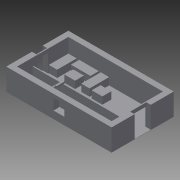
# Autodesk Inventor part: West_Structure_1st_Floor_CAFS
Saved by Autodesk Inventor 2014 (Build 180170000, 170)
## iProperties
Created: 2013-07-10
Part Number: West_Structure_1st_Floor_CAFS
Material: Generic
Document SubType Name: Modeling
Designer: jmw3
Density: 1 g/cm^3
Appearance: Default
Author: jmw3
Autodesk Inventor part; units mm, degrees
ref_plane "YZ Plane" through (0, 0, 0) normal (1, 0, 0) x (0, 1, 0)
ref_plane "XZ Plane" through (0, 0, 0) normal (0, 1, 0) x (-1, 0, 0)
ref_plane "XY Plane" through (0, 0, 0) normal (0, 0, 1) x (1, 0, 0)
sketch "Sketch1" plane through (0, 0, 0) normal (0, 0, 1) x (1, 0, 0)
  line L0 (-8321.04, 0) -> (8321.04, 0) projected
  line L1 (-5943.6, 3505.2) -> (5943.6, 3505.2)
  line L2 (-5334, 2895.6) -> (5334, 2895.6)
  line L3 (-4572, 2895.6) -> (-4419.6, 2895.6)
  line L4 (-1981.2, -2006.6) -> (-4445, -2006.6)
  line L5 (-4445, -2006.6) -> (-4445, -1892.3)
  line L6 (-1219.2, -2895.6) -> (-1066.8, -2895.6)
  line L7 (5334, -2895.6) -> (0, -2895.6)
  line L8 (0, -2895.6) -> (-5334, -2895.6)
  line L9 (5943.6, -3505.2) -> (0, -3505.2)
  line L10 (0, -3505.2) -> (-5943.6, -3505.2)
  line L11 (5334, 914.4) -> (5943.6, 914.4)
  line L12 (5943.6, -914.4) -> (5334, -914.4)
  line L13 (5334, 2895.6) -> (5334, 914.4)
  line L14 (5334, -914.4) -> (5334, -2895.6)
  line L15 (5943.6, 3505.2) -> (5943.6, 914.4)
  line L16 (5943.6, -914.4) -> (5943.6, -3505.2)
  line L17 (-4445, -2006.6) -> (5334, -2006.6)
  line L18 (5334, -1892.3) -> (-4445, -1892.3)
  line L19 (-4445, -1892.3) -> (-4445, -2006.6)
  line L20 (5334, -1892.3) -> (5334, -2006.6)
  line L21 (-5943.6, 609.6) -> (-5334, 609.6)
  line L22 (-5334, -609.6) -> (-5943.6, -609.6)
  line L23 (-5943.6, -3505.2) -> (-5943.6, -609.6)
  line L24 (-5943.6, 609.6) -> (-5943.6, 3505.2)
  line L25 (-5334, -2895.6) -> (-5334, -609.6)
  line L26 (-5334, 609.6) -> (-5334, 2895.6)
  line L27 (-4445, -2006.6) -> (-4419.6, -2006.6)
  line L28 (-4419.6, 2895.6) -> (-4572, 2895.6)
  line L29 (-4445, -1892.3) -> (-4445, -2006.6)
  line L30 (0, -4907.28) -> (0, 4907.28) projected
  dimension "d18" = 7010.4
  dimension "d19" = 609.6
  dimension "d20" = 609.6
  dimension "d23" = 1828.8
  dimension "d24" = 2590.8
  dimension "d25" = 609.6
  dimension "d28" = 114.3
  dimension "d29" = 0
  dimension "d34" = 1219.2
  dimension "d35" = 2895.6
  dimension "d36" = 609.6
  dimension "d46" = 889
  dimension "d105" = 889
  dimension "d106" = 11887.2
  constraints: 58 end point, 17 parallel, 8 horizontal, 7 collinear, 6 perpendicular, 4 point on line, 2 other
  measures "d18" distance between parallel lines of L10 L1
  measures "d19" distance between parallel lines of L10 L8
  measures "d20" distance between parallel lines of L1 L2
  measures "d23" distance between parallel lines of L12 L11
  measures "d24" distance between parallel lines of L9 L12
  measures "d25" distance between parallel lines of L15 L13
  measures "d28" distance between parallel lines of L17 L18
  measures "d29" distance between parallel lines of L13 L20
  measures "d34" distance between parallel lines of L22 L21
  measures "d35" distance between parallel lines of L10 L22
  measures "d36" distance between parallel lines of L24 L26
  measures "d46" distance between parallel lines of L26 L5
  measures "d105" distance from line of L6.end L17
  measures "d106" distance between parallel lines of L15 L24
extrude "Extrusion9" add sketch "Sketch1" along normal blind 2438.4 contours L18 L14 L17 L30 | L30 L17 L4 L5 L18 | L1 L30 L2 L26 L21 L24 | L1 L15 L11 L13 L2 L30 | L14 L12 L16 L9 L30 L7 | L30 L10 L23 L22 L25 L8 L6
sketch "Sketch8" plane through (0, 0, 0) normal (0, 0, -1) x (-1, 0, 0)
  line L0 (5943.6, 3505.2) -> (-5943.6, 3505.2) projected
  line L1 (-5943.6, 3505.2) -> (-5943.6, 914.4) projected
  line L2 (-5943.6, 914.4) -> (-5334, 914.4) projected
  line L3 (-5334, 914.4) -> (-5334, 2895.6) projected
  line L4 (-5334, 2895.6) -> (5334, 2895.6) projected
  line L5 (5334, 2895.6) -> (5334, 609.6) projected
  line L6 (5334, 609.6) -> (5943.6, 609.6) projected
  line L7 (5943.6, 609.6) -> (5943.6, 3505.2) projected
  line L8 (-5943.6, 3505.2) -> (5943.6, 3505.2)
  line L9 (5943.6, 3505.2) -> (5943.6, -3505.2)
  line L10 (5943.6, -3505.2) -> (-5943.6, -3505.2)
  line L11 (-5943.6, -3505.2) -> (-5943.6, 3505.2)
  point P0 (0, 0)
  constraints: 8 end point, 2 parallel, 1 horizontal, 1 perpendicular
extrude "Extrusion10" add sketch "Sketch8" along normal blind 25.4
sketch "Sketch10" plane through (-4445, -2006.6, 2438.4) normal (0, -1, 0) x (1, 0, 0)
  line L0 (0, -2438.4) -> (9779, -2438.4) projected
  line L1 (0, -2438.4) -> (0, 0) projected
  line L2 (723.9, -2438.4) -> (914.4, -2438.4)
  line L3 (914.4, -2438.4) -> (914.4, -2254.25)
  line L4 (914.4, -2254.25) -> (723.9, -2254.25)
  line L5 (723.9, -2254.25) -> (723.9, -2438.4)
  line L6 (914.4, -2254.25) -> (1104.9, -2254.25)
  line L7 (1104.9, -2254.25) -> (1104.9, -2070.1)
  line L8 (1104.9, -2070.1) -> (914.4, -2070.1)
  line L9 (914.4, -2070.1) -> (914.4, -2254.25)
  line L10 (1104.9, -2070.1) -> (1295.4, -2070.1)
  line L11 (1295.4, -2070.1) -> (1295.4, -1885.95)
  line L12 (1295.4, -1885.95) -> (1104.9, -1885.95)
  line L13 (1104.9, -1885.95) -> (1104.9, -2070.1)
  line L14 (1295.4, -1885.95) -> (1485.9, -1885.95)
  line L15 (1485.9, -1885.95) -> (1485.9, -1701.8)
  line L16 (1485.9, -1701.8) -> (1295.4, -1701.8)
  line L17 (1295.4, -1701.8) -> (1295.4, -1885.95)
  line L18 (1485.9, -1701.8) -> (1676.4, -1701.8)
  line L19 (1676.4, -1701.8) -> (1676.4, -1517.65)
  line L20 (1676.4, -1517.65) -> (1485.9, -1517.65)
  line L21 (1485.9, -1517.65) -> (1485.9, -1701.8)
  line L22 (1676.4, -1517.65) -> (1866.9, -1517.65)
  line L23 (1866.9, -1517.65) -> (1866.9, -1333.5)
  line L24 (1866.9, -1333.5) -> (1676.4, -1333.5)
  line L25 (1676.4, -1333.5) -> (1676.4, -1517.65)
  line L26 (1866.9, -1333.5) -> (2057.4, -1333.5)
  line L27 (2057.4, -1333.5) -> (2057.4, -1149.35)
  line L28 (2057.4, -1149.35) -> (1866.9, -1149.35)
  line L29 (1866.9, -1149.35) -> (1866.9, -1333.5)
  line L30 (2438.4, -965.2) -> (2438.4, -781.05)
  line L31 (2247.9, -1149.35) -> (2247.9, -965.2)
  line L32 (2247.9, -965.2) -> (2438.4, -965.2)
  line L33 (2438.4, -781.05) -> (2247.9, -781.05)
  line L34 (2247.9, -781.05) -> (2247.9, -965.2)
  line L35 (2057.4, -1149.35) -> (2247.9, -1149.35)
  line L36 (2247.9, -965.2) -> (2057.4, -965.2)
  line L37 (2057.4, -965.2) -> (2057.4, -1149.35)
  line L38 (2628.9, -781.05) -> (2628.9, -596.9)
  line L39 (2438.4, -781.05) -> (2628.9, -781.05)
  line L40 (2628.9, -596.9) -> (2438.4, -596.9)
  line L41 (2438.4, -596.9) -> (2438.4, -781.05)
  line L42 (3200.4, -228.6) -> (3200.4, -44.45)
  line L43 (3200.4, 139.7) -> (3200.4, -44.45)
  line L44 (3200.4, -44.45) -> (3390.9, -44.45)
  line L45 (3390.9, 139.7) -> (3200.4, 139.7)
  line L46 (3009.9, -44.45) -> (3009.9, -228.6)
  line L47 (3009.9, -228.6) -> (3200.4, -228.6)
  line L48 (3200.4, -44.45) -> (3009.9, -44.45)
  line L49 (3390.9, -44.45) -> (3390.9, 139.7)
  line L50 (3009.9, -412.75) -> (3009.9, -228.6)
  line L51 (3009.9, -228.6) -> (2819.4, -228.6)
  line L52 (2819.4, -412.75) -> (3009.9, -412.75)
  line L53 (2819.4, -228.6) -> (2819.4, -412.75)
  line L54 (2819.4, -596.9) -> (2819.4, -412.75)
  line L55 (2819.4, -412.75) -> (2628.9, -412.75)
  line L56 (2628.9, -596.9) -> (2819.4, -596.9)
  line L57 (2628.9, -412.75) -> (2628.9, -596.9)
  line L58 (3390.9, 139.7) -> (3581.4, 139.7)
  line L59 (3581.4, 139.7) -> (3581.4, 323.85)
  line L60 (3581.4, 323.85) -> (3390.9, 323.85)
  line L61 (3390.9, 323.85) -> (3390.9, 139.7)
  point P0 (8445.5, -2438.4)
  point P1 (4445, -2438.4)
  dimension "d113" = 190.5
  dimension "d115" = 184.15
  dimension "d116" = 723.9
  dimension "d117" = 190.5
  dimension "d118" = 184.15
  dimension "d119" = 190.5
  dimension "d120" = 184.15
  dimension "d121" = 190.5
  dimension "d122" = 184.15
  dimension "d123" = 190.5
  dimension "d124" = 184.15
  dimension "d125" = 190.5
  dimension "d126" = 184.15
  dimension "d127" = 190.5
  dimension "d128" = 184.15
  dimension "d129" = 190.5
  dimension "d130" = 184.15
  dimension "d131" = 190.5
  dimension "d132" = 184.15
  dimension "d133" = 190.5
  dimension "d134" = 184.15
  dimension "d135" = 190.5
  dimension "d136" = 184.15
  dimension "d137" = 190.5
  dimension "d138" = 184.15
  dimension "d139" = 190.5
  dimension "d140" = 184.15
  dimension "d141" = 190.5
  dimension "d142" = 184.15
  dimension "d154" = 184.15
  dimension "d155" = 190.5
  constraints: 120 end point, 30 parallel, 15 horizontal, 15 perpendicular, 12 collinear, 1 point on line
  measures "d113" distance between parallel lines of L3 L5
  measures "d115" distance between parallel lines of L4 L0
  measures "d116" distance between parallel lines of L1 L5
  measures "d117" distance between parallel lines of L9 L7
  measures "d118" distance between parallel lines of L8 L6
  measures "d119" distance between parallel lines of L11 L13
  measures "d120" distance between parallel lines of L12 L10
  measures "d121" distance between parallel lines of L17 L15
  measures "d122" distance between parallel lines of L16 L14
  measures "d123" distance between parallel lines of L19 L21
  measures "d124" distance between parallel lines of L20 L18
  measures "d125" distance between parallel lines of L25 L23
  measures "d126" distance between parallel lines of L24 L22
  measures "d127" distance between parallel lines of L27 L29
  measures "d128" distance between parallel lines of L28 L26
  measures "d129" distance between parallel lines of L37 L31
  measures "d130" distance between parallel lines of L36 L35
  measures "d131" distance between parallel lines of L30 L34
  measures "d132" distance between parallel lines of L33 L32
  measures "d133" distance between parallel lines of L38 L41
  measures "d134" distance between parallel lines of L40 L39
  measures "d135" distance between parallel lines of L57 L54
  measures "d136" distance between parallel lines of L55 L56
  measures "d137" distance between parallel lines of L50 L53
  measures "d138" distance between parallel lines of L51 L52
  measures "d139" distance between parallel lines of L46 L42
  measures "d140" distance between parallel lines of L48 L47
  measures "d141" distance between parallel lines of L49 L43
  measures "d142" distance between parallel lines of L45 L44
  measures "d154" distance between parallel lines of L58 L60
  measures "d155" distance between parallel lines of L61 L59
extrude "Stairs" add sketch "Sketch10" along normal up to surface (889 mm away)
sketch "Sketch9" plane through (0, 0, 2438.4) normal (0, 0, 1) x (1, 0, 0)
  line L0 (5943.6, 3505.2) -> (-5943.6, 3505.2) projected
  line L1 (-5943.6, 3505.2) -> (-5943.6, 609.6) projected
  line L2 (-5943.6, 609.6) -> (-5334, 609.6) projected
  line L3 (-5334, 609.6) -> (-5334, 2895.6) projected
  line L4 (-5334, 2895.6) -> (5334, 2895.6) projected
  line L5 (5334, 2895.6) -> (5334, 914.4) projected
  line L6 (5334, 914.4) -> (5943.6, 914.4) projected
  line L7 (5943.6, 914.4) -> (5943.6, 3505.2) projected
  line L8 (-5943.6, 609.6) -> (-5334, 609.6)
  line L9 (-5334, 609.6) -> (-5334, -609.6)
  line L10 (-5334, -609.6) -> (-5943.6, -609.6)
  line L11 (-5943.6, -609.6) -> (-5943.6, 609.6)
  line L12 (5334, 914.4) -> (5943.6, 914.4)
  line L13 (5943.6, 914.4) -> (5943.6, -914.4)
  line L14 (5943.6, -914.4) -> (5334, -914.4)
  line L15 (5334, -914.4) -> (5334, 914.4)
  line L16 (-5943.6, 609.6) -> (-5334, 609.6) projected
  line L17 (5334, 914.4) -> (5943.6, 914.4) projected
  line L18 (-5334, -609.6) -> (-5448.3, -609.6)
  line L19 (-5448.3, -609.6) -> (-5448.3, 609.6)
  line L20 (-5448.3, 609.6) -> (-5334, 609.6)
  line L21 (-5334, 609.6) -> (-5334, -609.6)
  line L22 (5334, -914.4) -> (5448.3, -914.4)
  line L23 (5448.3, -914.4) -> (5448.3, 914.4)
  line L24 (5448.3, 914.4) -> (5334, 914.4)
  line L25 (5334, 914.4) -> (5334, -914.4)
  point P0 (0, 0)
  dimension "d241" = 114.3
  dimension "d242" = 114.3
  constraints: 32 end point, 8 parallel, 4 horizontal, 4 perpendicular, 2 point on line
  measures "d241" distance between parallel lines of L21 L19
  measures "d242" distance between parallel lines of L25 L23
extrude "Doorways" add sketch "Sketch9" against normal blind 406.4 contours L23 L14 L15 L6 | L2 L9 L10 L19
sketch "Sketch11" plane through (-5943.6, -3505.2, 2438.4) normal (0, -1, 0) x (1, 0, 0)
  line L0 (5334, -406.4) -> (6553.2, -406.4)
  line L1 (6553.2, -406.4) -> (6553.2, -1625.6)
  line L2 (6553.2, -1625.6) -> (5334, -1625.6)
  line L3 (5334, -1625.6) -> (5334, -406.4)
  line L4 (11277.6, -2438.4) -> (2413, -2438.4) projected
  line L5 (5943.6, -2956.56) -> (5943.6, 492.76) projected
  point P0 (5943.6, -2438.4)
  dimension "d145" = 1219.2
  dimension "d147" = 1219.2
  dimension "d148" = 812.8
  constraints: 8 end point, 2 parallel, 1 horizontal, 1 perpendicular, 1 other
  measures "d145" distance between parallel lines of L0 L2
  measures "d147" distance between parallel lines of L1 L3
  measures "d148" distance between parallel lines of L4 L2
extrude "Window" cut sketch "Sketch11" against normal up to surface (609.6 mm away)
sketch "Furniture1" plane through (0, 0, 0) normal (0, 0, 1) x (1, 0, 0)
  line L0 (5334, 2895.6) -> (-5334, 2895.6) projected
  line L1 (-5334, 2895.6) -> (-5334, 609.6) projected
  line L2 (-5334, 2895.6) -> (-4394.2, 2895.6)
  line L3 (-4394.2, 2895.6) -> (-4394.2, 685.8)
  line L4 (-4394.2, 685.8) -> (-5334, 685.8)
  line L5 (-5334, 685.8) -> (-5334, 2895.6)
  line L6 (-4114.8, 2895.6) -> (-1905, 2895.6)
  line L7 (-1905, 2895.6) -> (-1905, 1955.8)
  line L8 (-1905, 1955.8) -> (-4114.8, 1955.8)
  line L9 (-4114.8, 1955.8) -> (-4114.8, 2895.6)
  line L10 (-1676.4, 2895.6) -> (-736.6, 2895.6)
  line L11 (-736.6, 2895.6) -> (-736.6, 685.8)
  line L12 (-736.6, 685.8) -> (-1676.4, 685.8)
  line L13 (-1676.4, 685.8) -> (-1676.4, 2895.6)
  line L14 (-3505.2, 1625.6) -> (-2305.2, 1625.6)
  line L15 (-2305.2, 1625.6) -> (-2305.2, 625.6)
  line L16 (-2305.2, 625.6) -> (-3505.2, 625.6)
  line L17 (-3505.2, 625.6) -> (-3505.2, 1625.6)
  line L18 (-431.8, 1625.6) -> (768.2, 1625.6)
  line L19 (768.2, 1625.6) -> (768.2, 625.6)
  line L20 (768.2, 625.6) -> (-431.8, 625.6)
  line L21 (-431.8, 625.6) -> (-431.8, 1625.6)
  point P0 (0, 0)
  dimension "d247" = 1000
  dimension "d248" = 1200
  dimension "d249" = 1000
  dimension "d250" = 1200
  dimension "d251" = 1270
  dimension "d252" = 1828.8
  dimension "d253" = 304.8
  dimension "d254" = 2209.8
  dimension "d255" = 939.8
  dimension "d256" = 939.8
  dimension "d257" = 939.8
  dimension "d258" = 2209.8
  dimension "d259" = 1219.2
  dimension "d260" = 3657.6
  constraints: 40 end point, 10 parallel, 5 horizontal, 5 perpendicular, 2 collinear, 2 point on line
  measures "d247" distance between parallel lines of L16 L14
  measures "d248" distance between parallel lines of L17 L15
  measures "d249" distance between parallel lines of L20 L18
  measures "d250" distance between parallel lines of L21 L19
  measures "d251" distance between parallel lines of L0 L14
  measures "d252" distance between parallel lines of L1 L17
  measures "d253" distance between parallel lines of L11 L21
  measures "d254" distance between parallel lines of L0 L4
  measures "d255" distance between parallel lines of L11 L13
  measures "d256" distance between parallel lines of L1 L3
  measures "d257" distance between parallel lines of L0 L8
  measures "d258" distance between parallel lines of L7 L9
  measures "d259" distance between parallel lines of L1 L9
  measures "d260" distance between parallel lines of L1 L13
extrude "Furniture+Pallets" add sketch "Furniture1" along normal blind 812.8
sketch "Instruments" plane through (0, 0, 0) normal (0, 0, 1) x (1, 0, 0)
  line L0 (5943.6, -914.4) -> (5334, -914.4) projected
  line L1 (5943.6, 914.4) -> (5334, 914.4) projected
  line L2 (-5334, 2895.6) -> (-5334, 609.6) projected
  line L3 (-5334, -609.6) -> (-5943.6, -609.6) projected
  line L4 (-8930.6312, 0) -> (8769.3036, 0) projected
  circle A0 centre (-1778, 0) radius 152.4
  circle A1 centre (1778, 0) radius 152.4
  circle A2 centre (-4889.5, -2451.1) radius 152.4
  line L5 (-5181.6, -152.4) -> (-5486.4, -152.4)
  line L6 (-5486.4, -152.4) -> (-5486.4, 152.4)
  line L7 (-5486.4, 152.4) -> (-5181.6, -152.4)
  line L8 (-5943.6, -3505.2) -> (-5943.6, 3505.2) projected
  line L9 (-5334, -609.6) -> (-5943.6, -609.6)
  line L10 (-5943.6, -609.6) -> (-5943.6, 609.6)
  line L11 (-5943.6, 609.6) -> (-5334, 609.6)
  line L12 (-5334, 609.6) -> (-5334, -609.6)
  line L13 (-5486.4, 609.6) -> (-5334, 609.6)
  line L14 (-5334, 609.6) -> (-5334, 457.2)
  line L15 (-5334, 457.2) -> (-5486.4, 457.2)
  line L16 (-5486.4, 457.2) -> (-5486.4, 609.6)
  line L17 (-5334, -609.6) -> (-5486.4, -609.6)
  line L18 (-5486.4, -609.6) -> (-5486.4, -457.2)
  line L19 (-5486.4, -457.2) -> (-5334, -457.2)
  line L20 (-5334, -457.2) -> (-5334, -609.6)
  line L21 (5943.6, 3505.2) -> (5943.6, -3505.2) projected
  line L22 (5486.4, 914.4) -> (5943.6, 914.4)
  line L23 (5943.6, 914.4) -> (5943.6, 1371.6)
  line L24 (5943.6, 1371.6) -> (5486.4, 1371.6)
  line L25 (5486.4, 1371.6) -> (5486.4, 914.4)
  line L26 (5943.6, -914.4) -> (5486.4, -914.4)
  line L27 (5486.4, -914.4) -> (5486.4, -1371.6)
  line L28 (5486.4, -1371.6) -> (5943.6, -1371.6)
  line L29 (5943.6, -1371.6) -> (5943.6, -914.4)
  line L30 (5486.4, 1371.6) -> (5943.6, 1371.6)
  line L31 (5943.6, 1371.6) -> (5943.6, -1371.6)
  line L32 (5943.6, -1371.6) -> (5486.4, -1371.6)
  line L33 (5334, 914.4) -> (5486.4, 914.4)
  line L34 (5486.4, 914.4) -> (5486.4, 0)
  line L35 (5486.4, 0) -> (5334, 0)
  line L36 (5334, 0) -> (5334, 914.4)
  line L37 (-5334, -2895.6) -> (-5334, 2895.6) projected
  line L38 (-1244.6, -2895.6) -> (-5334, -2895.6) projected
  line L39 (-5943.6, -609.6) -> (-5943.6, -3505.2) projected
  line L40 (-5943.6, -3505.2) -> (5943.6, -3505.2) projected
  line L41 (5943.6, -3505.2) -> (5943.6, -914.4) projected
  line L42 (5943.6, 3505.2) -> (-5943.6, 3505.2) projected
  line L43 (-5334, -2895.6) -> (-5334, 2895.6) projected
  line L44 (-5334, 2895.6) -> (5334, 2895.6) projected
  line L45 (5334, 2895.6) -> (5334, -1892.3) projected
  line L46 (5334, -1892.3) -> (-4445, -1892.3) projected
  line L47 (-4445, -1892.3) -> (-4445, -2006.6) projected
  line L48 (-4445, -2006.6) -> (-1244.6, -2006.6) projected
  line L49 (-1244.6, -2006.6) -> (-1054.1, -2006.6) projected
  line L50 (-1054.1, -2006.6) -> (5334, -2006.6) projected
  line L51 (5334, -2895.6) -> (-1054.1, -2895.6) projected
  line L52 (-1054.1, -2895.6) -> (-1244.6, -2895.6) projected
  line L53 (-1244.6, -2895.6) -> (-5334, -2895.6) projected
  line L54 (-5486.4, 457.2) -> (-5486.4, -457.2)
  line L55 (5486.4, 304.8) -> (5181.6, 304.8)
  line L56 (5181.6, 304.8) -> (5181.6, 609.6)
  line L57 (5486.4, 304.8) -> (5181.6, 609.6) construction
  line L58 (5181.6, 304.8) -> (5486.4, 609.6) construction
  line L59 (5181.6, 609.6) -> (5486.4, 304.8)
  line L60 (5486.4, -1371.6) -> (5486.4, 304.8)
  line L61 (5486.4, 609.6) -> (5486.4, 1371.6)
  line L62 (5181.6, -609.6) -> (5486.4, -609.6)
  line L63 (5181.6, -304.8) -> (5181.6, -609.6)
  line L64 (5181.6, -609.6) -> (5486.4, -304.8) construction
  line L65 (5486.4, -609.6) -> (5181.6, -304.8) construction
  line L66 (5181.6, -304.8) -> (5486.4, -609.6)
  line L67 (-5943.6, 3505.2) -> (-5943.6, 609.6) projected
  line L68 (-5943.6, 609.6) -> (-5448.3, 609.6) projected
  line L69 (5448.3, 914.4) -> (5943.6, 914.4) projected
  line L70 (5943.6, 914.4) -> (5943.6, 3505.2) projected
  line L71 (-5448.3, -609.6) -> (-5943.6, -609.6) projected
  line L72 (5943.6, -914.4) -> (5448.3, -914.4) projected
  line L73 (-5448.3, 609.6) -> (-5448.3, -609.6) projected
  line L74 (5448.3, -914.4) -> (5448.3, 914.4) projected
  line L75 (5334, -2006.6) -> (5334, -2895.6) projected
  point P0 (0, 0)
  point P1 (1.5875, 1.5875)
  point P2 (770.0638, -2405.9824)
  point P3 (-4729.4618, 0)
  point P4 (5334, 457.2)
  point P5 (5334, -457.2)
  dimension "d161" = 304.8
  dimension "d163" = 304.8
  dimension "d164" = 3556
  dimension "d165" = 7112
  dimension "d166" = 304.8
  dimension "d172" = 304.8
  dimension "d173" = 304.8
  dimension "d192" = 152.4
  dimension "d193" = 152.4
  dimension "d194" = 152.4
  dimension "d195" = 457.2
  dimension "d196" = 457.2
  dimension "d197" = 457.2
  dimension "d198" = 457.2
  dimension "d227" = 444.5
  dimension "d228" = 444.5
  dimension "d229" = 152.4
  dimension "d230" = 152.4
  dimension "d231" = 457.2
  dimension "d234" = 304.8
  dimension "d235" = 304.8
  dimension "d236" = 152.4
  dimension "d237" = 304.8
  dimension "d238" = 304.8
  dimension "d239" = 152.4
  dimension "d240" = 457.2
  constraints: 86 end point, 17 parallel, 11 point on line, 9 horizontal, 8 perpendicular, 4 midpoint, 3 centre point, 3 collinear, 1 coincident
  measures "d161" diameter of A1
  measures "d163" diameter of A0
  measures "d164" distance from line of L2 A0.centre
  measures "d165" distance from line of L2 A1.centre
  measures "d166" diameter of A2
  measures "d172" distance of L5.start L5.end
  measures "d173" distance of L5.end L6.end
  measures "d192" distance between parallel lines of L14 L16
  measures "d193" distance between parallel lines of L13 L15
  measures "d194" distance between parallel lines of L3 L19
  measures "d195" distance between parallel lines of L22 L24
  measures "d196" distance between parallel lines of L25 L21
  measures "d197" distance between parallel lines of L27 L29
  measures "d198" distance between parallel lines of L0 L28
  measures "d227" distance from line of L38 A2.centre
  measures "d228" distance from line of L37 A2.centre
  measures "d229" distance between parallel lines of L12 L6
  measures "d230" distance between parallel lines of L4 L5
  measures "d231" distance from line of L1 point (5334, 457.2)
  measures "d234" distance of L55.end L56.end
  measures "d235" distance of L55.start L55.end
  measures "d236" distance between parallel lines of L36 L56
  measures "d237" distance of L62.start L62.end
  measures "d238" distance of L63.start L62.start
  measures "d239" distance between parallel lines of L45 L63
  measures "d240" distance from line of L0 point (5334, -457.2)
sketch "Furniture2" plane through (0, 0, 0) normal (0, 0, 1) x (1, 0, 0)
  line L0 (5334, 2895.6) -> (-5334, 2895.6) projected
  line L1 (-5334, 2895.6) -> (-4394.2, 2895.6)
  line L2 (-4394.2, 2895.6) -> (-4394.2, 685.8)
  line L3 (-4394.2, 685.8) -> (-5334, 685.8)
  line L4 (-5334, 685.8) -> (-5334, 2895.6)
  line L5 (-3175, 2895.6) -> (-2235.2, 2895.6)
  line L6 (-2235.2, 2895.6) -> (-2235.2, 685.8)
  line L7 (-2235.2, 685.8) -> (-3175, 685.8)
  line L8 (-3175, 685.8) -> (-3175, 2895.6)
  line L9 (-76.2, 2895.6) -> (-76.2, 685.8)
  line L10 (-76.2, 685.8) -> (-1016, 685.8)
  line L11 (-1016, 2895.6) -> (-76.2, 2895.6)
  line L12 (-1016, 685.8) -> (-1016, 2895.6)
  point P0 (0, 0)
  dimension "d261" = 2209.8
  dimension "d262" = 939.8
  dimension "d263" = 2209.8
  dimension "d264" = 939.8
  dimension "d265" = 2209.8
  dimension "d266" = 939.8
  dimension "d267" = 1219.2
  dimension "d268" = 1219.2
  constraints: 24 end point, 6 parallel, 3 horizontal, 3 perpendicular, 2 collinear
  measures "d261" distance between parallel lines of L1 L3
  measures "d262" distance between parallel lines of L4 L2
  measures "d263" distance between parallel lines of L5 L7
  measures "d264" distance between parallel lines of L8 L6
  measures "d265" distance between parallel lines of L11 L10
  measures "d266" distance between parallel lines of L12 L9
  measures "d267" distance between parallel lines of L2 L8
  measures "d268" distance between parallel lines of L6 L12
body "Solid2"
